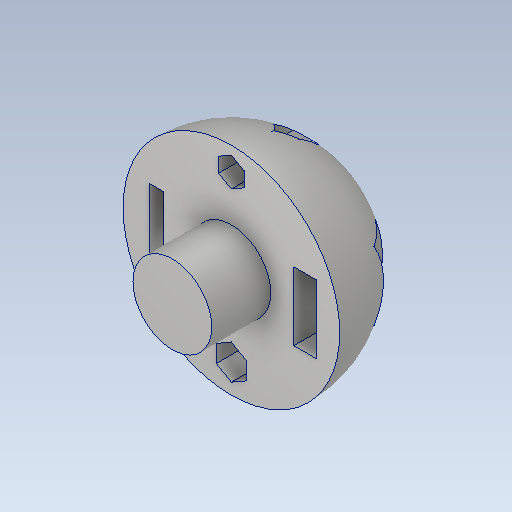
# Autodesk Inventor part: Rotatory Hinge 1_CPY
Saved by Autodesk Inventor 2021 (Build 250183000, 183)
## iProperties
Created: 2021-03-10
Part Number: Rotatory Hinge 1_CPY
Material: Aluminum 6061
Document SubType Name: Modeling
Designer: 91730
Density: 2.7 g/cm^3
Appearance: Aluminum - Flat
Author: Asus
Autodesk Inventor part; units mm, degrees
ref_plane "YZ Plane" through (0, 0, 0) normal (1, 0, 0) x (0, 1, 0)
ref_plane "XZ Plane" through (0, 0, 0) normal (0, 1, 0) x (-1, 0, 0)
ref_plane "XY Plane" through (0, 0, 0) normal (0, 0, 1) x (1, 0, 0)
sketch "Sketch1" plane through (0, 0, 0) normal (0, 0, 1) x (1, 0, 0)
  arc A0 (55, 0) -> (-55, 0) centre (0, 0) ccw
  line L0 (-55, 0) -> (55, 0)
  dimension "d0" = 55
  dimension "d1" = 110
  constraints: 2 end point, 2 point on circle, 1 centre point, 1 coincident, 1 horizontal
  measures "d0" radius of A0
  measures "d1" distance of L0.start L0.end
revolve "Revolution1" add sketch "Sketch1" angle 180 about axis through (-55, 0, 0) along (-1, 0, 0)
sketch "Sketch2" plane through (0, 0, 0) normal (0, 0, 1) x (1, 0, 0)
  circle A0 centre (0, 0) radius 20
  dimension "d9" = 40
  constraints: 1 centre point, 1 coincident
  measures "d9" diameter of A0
sketch "Sketch3" plane through (0, 0, 0) normal (0, 0, 1) x (1, 0, 0)
  line L0 (-34.2608, -17.3432) -> (-41.496, -17.3432)
  line L1 (-41.496, -17.3432) -> (-41.496, 17.3432)
  line L2 (-41.496, 17.3432) -> (-34.2608, 17.3432)
  line L3 (-34.2608, 17.3432) -> (-34.2608, -17.3432)
  line L4 (-34.2608, -17.3432) -> (-41.496, 17.3432) construction
  line L5 (-41.496, -17.3432) -> (-34.2608, 17.3432) construction
  line L6 (43.1984, -17.3432) -> (31.7072, -17.3432)
  line L7 (31.7072, -17.3432) -> (31.7072, 17.3432)
  line L8 (31.7072, 17.3432) -> (43.1984, 17.3432)
  line L9 (43.1984, 17.3432) -> (43.1984, -17.3432)
  line L10 (43.1984, -17.3432) -> (31.7072, 17.3432) construction
  line L11 (31.7072, -17.3432) -> (43.1984, 17.3432) construction
  point P0 (0, 0)
  point P1 (-37.8784, 0)
  point P2 (37.4528, 0)
  constraints: 24 end point, 4 midpoint, 4 parallel, 2 horizontal, 2 perpendicular, 1 point on line
extrude "Extrusion1" cut sketch "Sketch3" against normal blind 55
sketch "Sketch4" plane through (0, 0, 0) normal (0, 0, 1) x (1, 0, 0)
  line L0 (0, 35.7372) -> (-6.4528, 39.4627)
  line L1 (-6.4528, 39.4627) -> (-6.4528, 46.9137)
  line L2 (-6.4528, 46.9137) -> (0, 50.6392)
  line L3 (0, 50.6392) -> (6.4528, 46.9137)
  line L4 (6.4528, 46.9137) -> (6.4528, 39.4627)
  line L5 (6.4528, 39.4627) -> (0, 35.7372)
  line L6 (0, -31.5978) -> (7.6477, -36.0132)
  line L7 (7.6477, -36.0132) -> (7.6477, -44.844)
  line L8 (7.6477, -44.844) -> (0, -49.2594)
  line L9 (0, -49.2594) -> (-7.6477, -44.844)
  line L10 (-7.6477, -44.844) -> (-7.6477, -36.0132)
  line L11 (-7.6477, -36.0132) -> (0, -31.5978)
  point P0 (0, 0)
  point P1 (0, 43.1882)
  point P2 (0, -40.4286)
  constraints: 24 end point, 26 other
extrude "Extrusion2" cut sketch "Sketch4" against normal blind 55
extrude "Extrusion4" add sketch "Sketch2" along normal blind 30
body "Solid1"
